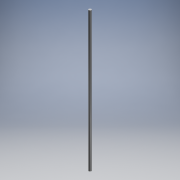
# Autodesk Inventor part: 8mm hardened rod
Saved by Autodesk Inventor 2017 (Build 210142000, 142)
## iProperties
Part Number: 8mm hardened rod
Material: Edelstahl, 440C
Document SubType Name: Modeling
Designer: Till
Density: 7.75 g/cm^3
Appearance: Edelstahl - hell
Author: Till
Autodesk Inventor part; units mm, degrees
ref_plane "YZ Plane" through (0, 0, 0) normal (1, 0, 0) x (0, 1, 0)
ref_plane "XZ Plane" through (0, 0, 0) normal (0, 1, 0) x (-1, 0, 0)
ref_plane "XY Plane" through (0, 0, 0) normal (0, 0, 1) x (1, 0, 0)
sketch "Skizze1" plane through (0, 0, 0) normal (0, 0, 1) x (1, 0, 0)
  circle A0 centre (0, 0) radius 4
  dimension "d0" = 8
  constraints: 1 centre point, 1 coincident
  measures "d0" diameter of A0
extrude "Extrusion1" add sketch "Skizze1" along normal blind 440
